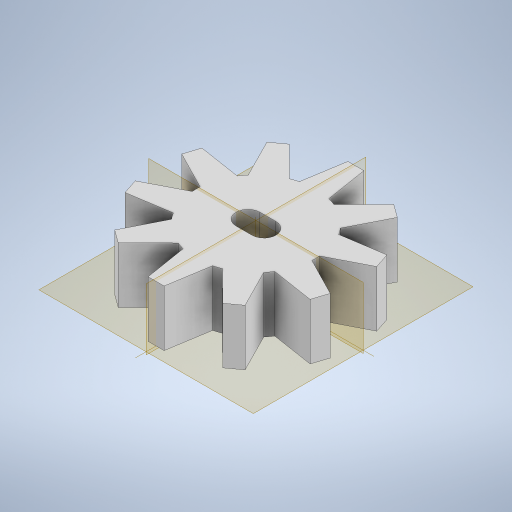
# Autodesk Inventor part: zahnrad
Saved by Autodesk Inventor 2023 (Build 270158000, 158)
## iProperties
Created: 2022-06-29
Part Number: zahnrad
Material: Generic
Document SubType Name: Modeling
Designer: Habib
Density: 1 g/cm^3
Appearance: Default
Author: Habib
Autodesk Inventor part; units mm, degrees
sketch "Sketch1" plane through (0, 0, 0) normal (0, 1, 0) x (-1, 0, 0)
  circle A0 centre (0, 0) radius 7.5
  dimension "d0" = 15
  constraints: 1 centre point, 1 coincident
  measures "d0" diameter of A0
extrude "Extrusion1" add sketch "Sketch1" along normal blind 7
sketch "Sketch2" plane through (0, 7, 0) normal (0, 1, 0) x (1, 0, 0)
  line L0 (0, 0) -> (2.5, 0)
  line L1 (2.5, 0) -> (-2.5, 0) construction
  line L2 (1, 1.5) -> (-1, 1.5)
  line L3 (-1, -1.5) -> (1, -1.5)
  arc A0 (1, -1.5) -> (1, 1.5) centre (1, 0) ccw
  arc A1 (-1, 1.5) -> (-1, -1.5) centre (-1, 0) ccw
  dimension "d3" = 2.5
  dimension "d4" = 5
  dimension "d5" = 3
  constraints: 10 end point, 6 point on circle, 4 tangent, 2 centre point, 2 horizontal, 2 point on line, 1 midpoint, 1 parallel
  measures "d3" distance of L0.start L0.end
  measures "d4" distance of L0.end L1.end
  measures "d5" diameter of A1
extrude "Extrusion2" cut sketch "Sketch2" against normal blind 7
sketch "Sketch3" plane through (0, 0, 0) normal (0, 1, 0) x (-1, 0, 0)
  circle A0 centre (0, 0) radius 7.5 projected
  line L0 (0, 12.5) -> (1, 12.5)
  line L1 (1, 12.5) -> (1.844, 7.2698)
  line L2 (-1, 12.5) -> (-1.844, 7.2698)
  line L3 (0, 12.5) -> (-1, 12.5)
  line L4 (-7.3473, 10.1127) -> (-6.5383, 10.7005)
  line L5 (-7.3473, 10.1127) -> (-8.1563, 9.5249)
  line L6 (-8.1563, 9.5249) -> (-5.7649, 4.7975)
  line L7 (-6.5383, 10.7005) -> (-2.7813, 6.9652)
  line L8 (-11.8882, 3.8627) -> (-11.5792, 4.8138)
  line L9 (-11.8882, 3.8627) -> (-12.1972, 2.9117)
  line L10 (-12.1972, 2.9117) -> (-7.4838, 0.4928)
  line L11 (-11.5792, 4.8138) -> (-6.3442, 4.0002)
  line L12 (-11.8882, -3.8627) -> (-12.1972, -2.9117)
  line L13 (-11.8882, -3.8627) -> (-11.5792, -4.8138)
  line L14 (-11.5792, -4.8138) -> (-6.3442, -4.0002)
  line L15 (-12.1972, -2.9117) -> (-7.4838, -0.4928)
  line L16 (-7.3473, -10.1127) -> (-8.1563, -9.5249)
  line L17 (-7.3473, -10.1127) -> (-6.5383, -10.7005)
  line L18 (-6.5383, -10.7005) -> (-2.7813, -6.9652)
  line L19 (-8.1563, -9.5249) -> (-5.7649, -4.7975)
  line L20 (0, -12.5) -> (-1, -12.5)
  line L21 (0, -12.5) -> (1, -12.5)
  line L22 (1, -12.5) -> (1.844, -7.2698)
  line L23 (-1, -12.5) -> (-1.844, -7.2698)
  line L24 (7.3473, -10.1127) -> (6.5383, -10.7005)
  line L25 (7.3473, -10.1127) -> (8.1563, -9.5249)
  line L26 (8.1563, -9.5249) -> (5.7649, -4.7975)
  line L27 (6.5383, -10.7005) -> (2.7813, -6.9652)
  line L28 (11.8882, -3.8627) -> (11.5792, -4.8138)
  line L29 (11.8882, -3.8627) -> (12.1972, -2.9117)
  line L30 (12.1972, -2.9117) -> (7.4838, -0.4928)
  line L31 (11.5792, -4.8138) -> (6.3442, -4.0002)
  line L32 (11.8882, 3.8627) -> (12.1972, 2.9117)
  line L33 (11.8882, 3.8627) -> (11.5792, 4.8138)
  line L34 (11.5792, 4.8138) -> (6.3442, 4.0002)
  line L35 (12.1972, 2.9117) -> (7.4838, 0.4928)
  line L36 (7.3473, 10.1127) -> (8.1563, 9.5249)
  line L37 (7.3473, 10.1127) -> (6.5383, 10.7005)
  line L38 (6.5383, 10.7005) -> (2.7813, 6.9652)
  line L39 (8.1563, 9.5249) -> (5.7649, 4.7975)
  dimension "d9" = 1
  dimension "d12" = 360
  constraints: 80 end point, 1 horizontal, 93 other
  measures "d9" distance of L0.start L0.end
extrude "Extrusion3" add sketch "Sketch3" along normal blind 7 contours A0 L34 L33 L32 L35 | L30 L29 L28 L31 A0 | A0 L38 L37 L36 L39 | L26 L25 L24 L27 A0 | A0 L2 L3 L0 L1 | L22 L21 L20 L23 A0 | A0 L6 L5 L4 L7 | L18 L17 L16 L19 A0 | A0 L10 L9 L8 L11 | L14 L13 L12 L15 A0
body "Solid1"
